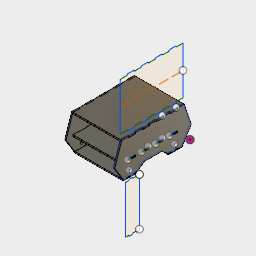
Phantom Chassis v1 (Autodesk Fusion 360 design; units mm, degrees)
Autodesk Fusion 360 part; units mm, degrees
note: some values were not read from the file. Set by a fixed rule: which sketch regions a step uses.
sketch "Sketch1" plane through (0, 0, 0) normal (1, 0, 0) x (0, 1, 0)
  line L0 (-200, 100) -> (-220, 40)
  line L1 (-195, 0) -> (-220, 40)
  line L2 (-25, 0) -> (0, 40)
  line L3 (0, 40) -> (-20, 100)
  line L4 (-65, 0) -> (-85, 15)
  line L5 (-85, 15) -> (-135, 15)
  line L6 (-135, 15) -> (-155, 0)
  line L7 (-179.9981, 100) -> (-179.9981, 97)
  line L8 (-160, 97) -> (-160, 100)
  line L9 (-179.9981, 100) -> (-179.9981, 97)
  line L10 (-160, 97) -> (-160, 100)
  line L11 (-160, 100) -> (-140, 100)
  line L12 (-140, 100) -> (-140, 97)
  line L13 (-20, 100) -> (-40, 100)
  line L14 (-40, 100) -> (-40, 97)
  line L15 (-60, 97) -> (-60, 100)
  line L16 (-40, 100) -> (-40, 97)
  line L17 (-60, 100) -> (-80, 100)
  line L18 (-80, 100) -> (-80, 97)
  line L19 (-60, 97) -> (-60, 100)
  line L20 (-140, 97) -> (-140, 100)
  line L21 (-80, 100) -> (-80, 97)
  line L22 (-40, 100) -> (-20, 100)
  line L23 (-80, 100) -> (-60, 100)
  line L24 (-200, 100) -> (-179.9981, 100)
  line L25 (-160, 100) -> (-140, 100)
  line L26 (-160, 97) -> (-179.9981, 97)
  line L27 (-40, 97) -> (-60, 97)
  line L28 (-120, 96.9801) -> (-120, 100)
  line L29 (-120, 96.9801) -> (-140, 97)
  line L30 (-65, 0) -> (-55, 0)
  line L31 (-25, 0) -> (-25, -3)
  line L32 (-25, -3) -> (-35, -3)
  line L33 (-35, 0) -> (-35, -3)
  line L34 (-45, -3) -> (-45, 0)
  line L35 (-55, -3) -> (-55, 0)
  line L36 (-35, 0) -> (-45, 0)
  line L37 (-55, 0) -> (-65, 0)
  line L38 (-35, 0) -> (-45, 0)
  line L39 (-55, 0) -> (-65, 0)
  line L40 (-55, -3) -> (-45, -3)
  line L41 (-195, 0) -> (-195, -3)
  line L42 (-195, -3) -> (-185, -3)
  line L43 (-185, -3) -> (-185, 0)
  line L44 (-175, 0) -> (-175, -3)
  line L45 (-175, -3) -> (-165, -3)
  line L46 (-165, -3) -> (-165, 0)
  line L47 (-180, 40) -> (-180, 43)
  line L48 (-140, 43) -> (-140, 40)
  line L49 (-100, 43) -> (-100, 40)
  line L50 (-120, 40) -> (-120, 44)
  line L51 (-60, 43) -> (-60, 40)
  line L52 (-80, 40) -> (-80, 44)
  line L53 (-40, 43) -> (-40, 40)
  line L54 (-155, 0) -> (-165, 0)
  line L55 (-175, 0) -> (-185, 0)
  line L56 (-185, 0) -> (-175, 0)
  line L57 (-165, 0) -> (-155, 0)
  line L58 (-120, 100) -> (-100, 100)
  line L59 (-80, 97) -> (-100, 97)
  line L60 (-100, 97) -> (-100, 100)
  line L61 (-180, 43) -> (-160, 43)
  line L62 (-160, 43) -> (-160, 40)
  line L63 (-160, 40) -> (-180, 40)
  line L64 (-180, 40) -> (-180, 43)
  line L65 (-140, 43) -> (-120, 43)
  line L66 (-120, 43) -> (-120, 40)
  line L67 (-120, 40) -> (-140, 40)
  line L68 (-140, 40) -> (-140, 43)
  line L69 (-100, 43) -> (-80, 43)
  line L70 (-80, 43) -> (-80, 40)
  line L71 (-80, 40) -> (-100, 40)
  line L72 (-100, 40) -> (-100, 43)
  line L73 (-60, 43) -> (-40, 43)
  line L74 (-40, 43) -> (-40, 40)
  line L75 (-40, 40) -> (-60, 40)
  line L76 (-60, 40) -> (-60, 43)
  circle A0 centre (-175, 12) radius 4
  circle A1 centre (-45, 12) radius 4
  dimension "d22" = 3
  dimension "d23" = 3
  dimension "d25" = 3
  dimension "d26" = 3
  dimension "d27" = 3
  dimension "d28" = 3
  dimension "d29" = 3
  dimension "d30" = 3
  dimension "d42" = 3
  constraint horizontal L24
  constraint coincident origin L24
  constraint coincident origin L38
  constraint vertical L7
  constraint vertical L8
  constraint vertical L9
  constraint vertical L10
  constraint horizontal L11
  constraint vertical L12
  constraint vertical L14
  constraint vertical L15
  constraint vertical L16
  constraint vertical L19
  constraint vertical L20
  constraint collinear L24 L25
  constraint coincident L27
  constraint perpendicular L31 L32
  constraint perpendicular L32 L33
  constraint perpendicular L34 L36
  constraint perpendicular L33 L38
  constraint perpendicular L34 L40
  constraint perpendicular L41 L54
  constraint perpendicular L41 L42
  constraint coincident origin L54
  constraint perpendicular L44 L54
  constraint perpendicular L44 L45
  constraint coincident origin L56
  constraint vertical L47
  constraint vertical L48
  constraint vertical L49
  constraint vertical L50
  constraint vertical L51
  constraint vertical L52
  constraint vertical L53
  constraint collinear L54 L55
  constraint collinear L56 L57
  constraint perpendicular L28 L58
  constraint perpendicular L18 L59
  constraint perpendicular L58 L60
  constraint horizontal L61
  constraint vertical L62
  constraint horizontal L63
  constraint vertical L64
  constraint horizontal L65
  constraint vertical L66
  constraint horizontal L67
  constraint vertical L68
  constraint horizontal L69
  constraint vertical L70
  constraint horizontal L71
  constraint vertical L72
  constraint horizontal L73
  constraint vertical L74
  constraint horizontal L75
  constraint vertical L76
  constraint perpendicular L30 L35
  constraint collinear L17 L58
  constraint collinear L13 L17
  measures "d42" distance of origin
sketch "Sketch3" plane through (0, 0, 0) normal (1, 0, 0) x (0, 1, 0)
  line L0 (-175, -11) -> (-165, -11)
  line L1 (-165, -11) -> (-165, -14)
  line L2 (-175, -14) -> (-175, -11)
  line L3 (-155, -11) -> (-145, -11)
  line L4 (-145, -11) -> (-145, -14)
  line L5 (-155, -14) -> (-155, -11)
  line L6 (-145, -14) -> (-145, -153)
  line L7 (-185, -150) -> (-185, -14)
  line L8 (-175, -153) -> (-165, -153)
  line L9 (-165, -153) -> (-165, -150)
  line L10 (-175, -150) -> (-175, -153)
  line L11 (-145, -150) -> (-145, -153)
  line L12 (-145, -153) -> (-155, -153)
  line L13 (-155, -153) -> (-155, -150)
  line L14 (-175, -150) -> (-185, -150)
  line L15 (-165, -150) -> (-155, -150)
  line L16 (-145, -153) -> (-155, -153)
  line L17 (-165, -153) -> (-175, -153)
  line L18 (-185, -14) -> (-175, -14)
  line L19 (-165, -14) -> (-155, -14)
  dimension "d39" = 3
  dimension "d40" = 3
  dimension "d41" = 3
  constraint horizontal L0
  constraint vertical L1
  constraint vertical L2
  constraint horizontal L3
  constraint vertical L4
  constraint vertical L5
  constraint horizontal L18
  constraint vertical L6
  constraint horizontal L16
  constraint vertical L7
  constraint horizontal L8
  constraint vertical L9
  constraint vertical L10
  constraint vertical L11
  constraint horizontal L12
  constraint vertical L13
  constraint perpendicular L7 L14
  constraint perpendicular L9 L15
  constraint collinear L16 L17
  constraint collinear L18 L19
sketch "Sketch4" plane through (0, 0, 0) normal (1, 0, 0) x (0, 1, 0)
  line L0 (-20, 115) -> (-20, 250)
  line L1 (-40, 111) -> (-60, 111)
  line L2 (-60, 111) -> (-40, 111)
  line L3 (-20, 114) -> (-20, 115)
  line L4 (-20, 114) -> (-40, 114)
  line L5 (-40, 114) -> (-40, 111)
  line L6 (-60, 111) -> (-60, 114)
  line L7 (-60, 114) -> (-80, 114)
  line L8 (-80, 114) -> (-80, 111)
  line L9 (-80, 111) -> (-100, 111)
  line L10 (-100, 111) -> (-100, 114)
  line L11 (-100, 114) -> (-120, 114)
  line L12 (-120, 114) -> (-120, 111)
  line L13 (-120, 111) -> (-140, 111)
  line L14 (-140, 111) -> (-140, 114)
  line L15 (-140, 114) -> (-160, 114)
  line L16 (-160, 114) -> (-160, 111)
  line L17 (-160, 111) -> (-180, 111)
  line L18 (-180, 111) -> (-180, 114)
  line L19 (-180, 114) -> (-200, 114)
  line L20 (-200, 114) -> (-200, 250)
  line L21 (-20, 250) -> (-40, 250)
  line L22 (-40, 250) -> (-40, 253)
  line L23 (-40, 253) -> (-60, 253)
  line L24 (-60, 253) -> (-60, 250)
  line L25 (-60, 250) -> (-80, 250)
  line L26 (-80, 250) -> (-80, 253)
  line L27 (-80, 253) -> (-100, 253)
  line L28 (-100, 253) -> (-100, 250)
  line L29 (-100, 250) -> (-120, 250)
  line L30 (-120, 250) -> (-120, 253)
  line L31 (-120, 253) -> (-140, 253)
  line L32 (-140, 253) -> (-140, 250)
  line L33 (-140, 250) -> (-160, 250)
  line L34 (-160, 250) -> (-160, 253)
  line L35 (-160, 253) -> (-180, 253)
  line L36 (-180, 253) -> (-180, 250)
  line L37 (-180, 250) -> (-200, 250)
  line L38 (-200, 182) -> (-20, 182) construction
  dimension "d31" = 3
  dimension "d32" = 3
  dimension "d33" = 3
  dimension "d34" = 3
  dimension "d35" = 3
  dimension "d36" = 3
  dimension "d37" = 3
  dimension "d38" = 3
  constraint vertical L0
  constraint horizontal L1
  constraint parallel L0 L3
  constraint perpendicular L3 L4
  constraint perpendicular L1 L5
  constraint perpendicular L1 L6
  constraint perpendicular L6 L7
  constraint parallel L6 L8
  constraint perpendicular L8 L9
  constraint perpendicular L9 L10
  constraint perpendicular L10 L11
  constraint perpendicular L11 L12
  constraint perpendicular L12 L13
  constraint perpendicular L13 L14
  constraint perpendicular L14 L15
  constraint perpendicular L15 L16
  constraint perpendicular L14 L17
  constraint perpendicular L17 L18
  constraint perpendicular L19 L20
  constraint perpendicular L0 L21
  constraint perpendicular L21 L22
  constraint perpendicular L22 L23
  constraint perpendicular L21 L24
  constraint perpendicular L22 L25
  constraint perpendicular L21 L26
  constraint perpendicular L26 L27
  constraint perpendicular L27 L28
  constraint perpendicular L28 L29
  constraint perpendicular L29 L30
  constraint perpendicular L30 L31
  constraint perpendicular L31 L32
  constraint perpendicular L32 L33
  constraint perpendicular L33 L34
  constraint perpendicular L32 L35
  constraint perpendicular L35 L36
  constraint perpendicular L20 L37
  constraint midpoint L20 origin
  measures "d31" distance of origin
  measures "d32" distance of origin
  measures "d33" distance of origin
  measures "d34" distance of origin
  measures "d35" distance of origin
  measures "d36" distance of origin
  measures "d37" distance of origin
  measures "d38" distance of origin
extrude "Extrude1" add sketch "Sketch4" along normal blind 4 makes body 1
extrude "Extrude2" add sketch "Sketch1" along normal blind 4 separate body makes body 2
extrude "Extrude3" add sketch "Sketch3" along normal blind 4 separate body makes body 3
extrude "Extrude4" add sketch "Sketch4" along normal blind 4 separate body makes body 4
extrude "Extrude5" add sketch "Sketch1" along normal blind 4 separate body makes body 5
extrude "Extrude6" add sketch "Sketch3" along normal blind 4 separate body makes body 6
move_body "MoveBody1" bodies 4 to x (0, 0, 1) y (0, 1, 0) z (-1, 0, 0) at (157.1293, 0, 157.1293)
move_body "MoveBody2" bodies 1 to x (0, 0, -1) y (0, 1, 0) z (1, 0, 0) at (-198.7281, 0, 206.7281)
move_body "MoveBody3" bodies 6 to x (0, 0, -1) y (0, 1, 0) z (1, 0, 0) at (44.7719, 0, -44.7719)
move_body "MoveBody4" bodies 3 to x (0, 0, -1) y (0, 1, 0) z (1, 0, 0) at (91.1516, 0, -91.1516)
move_body "MoveBody5" bodies 6 to x (1, 0, 0) y (0, 1, 0) z (0, 0, 1) at (0, -10, 45)
move_body "MoveBody6" bodies 6 to x (1, 0, 0) y (0, 1, 0) z (0, 0, 1) at (0, 0, -0.25)
move_body "MoveBody7" bodies 6 to x (1, 0, 0) y (0, 1, 0) z (0, 0, 1) at (-30.8, 0, 0)
move_body "MoveBody8" bodies 4 to x (1, 0, 0) y (0, 1, 0) z (0, 0, 1) at (-43, 0, -117)
move_body "MoveBody9" bodies 3 to x (1, 0, 0) y (0, 1, 0) z (0, 0, 1) at (-77.2, 0, 90)
move_body "MoveBody10" bodies 3 to x (1, 0, 0) y (0, 1, 0) z (0, 0, 1) at (0, 0, 1.1)
move_body "MoveBody11" bodies 3 to x (1, 0, 0) y (0, 1, 0) z (0, 0, 1) at (0, 120, 0)
move_body "MoveBody12" bodies 3 to x (1, 0, 0) y (0, 1, 0) z (0, 0, 1) at (0, 0, 0.05)
move_body "MoveBody13" bodies 3 to x (1, 0, 0) y (0, 1, 0) z (0, 0, 1) at (0.05, 0, 0)
move_body "MoveBody14" bodies 6 to x (1, 0, 0) y (0, 1, 0) z (0, 0, 1) at (0, 0, 0.02)
move_body "MoveBody15" bodies 5 to x (1, 0, 0) y (0, 1, 0) z (0, 0, 1) at (-140.05, 0, 0)
move_body "MoveBody16" bodies 1 to x (1, 0, 0) y (0, 1, 0) z (0, 0, 1) at (-51.2, 0, -106.7)
move_body "MoveBody17" bodies 3 to x (1, 0, 0) y (0, -1, 0) z (0, 0, -1) at (0, -116.1802, -8.0033)
move_body "MoveBody18" bodies 3 to x (1, 0, 0) y (0, 1, 0) z (0, 0, 1) at (0, 26, 4)
move_body "MoveBody19" bodies 3 to x (1, 0, 0) y (0, 1, 0) z (0, 0, 1) at (0, 0.2, 0)
move_body "MoveBody20" bodies 5 to x (1, 0, 0) y (0, 1, 0) z (0, 0, 1) at (0.12, 0, 0.04)
move_body "MoveBody21" bodies 6 to x (1, 0, 0) y (0, 1, 0) z (0, 0, 1) at (0.1, 0, 0.05)
move_body "MoveBody22" bodies 6 to x (1, 0, 0) y (0, 1, 0) z (0, 0, 1) at (0, 0, -0.01)
move_body "MoveBody23" bodies 3 to x (1, 0, 0) y (0, 1, 0) z (0, 0, 1) at (0.07, 0, 0)
move_body "MoveBody24" bodies 3 to x (1, 0, 0) y (0, 1, 0) z (0, 0, 1) at (0, 0, 0.04)
move_body "MoveBody25" bodies 2 to x (1, 0, 0) y (0, 1, 0) z (0, 0, 1) at (0.07, 0, 0)
move_body "MoveBody26" bodies 2 to x (1, 0, 0) y (0, 1, 0) z (0, 0, 1) at (0.002, 0, 0)
move_body "MoveBody27" bodies 2 to x (1, 0, 0) y (0, 1, 0) z (0, 0, 1) at (0, 0, 0.038)
equation "thick = 3 mm"
equation "d22 = thick"
equation "d23 = thick"
equation "d25 = thick"
equation "d26 = thick"
equation "d27 = thick"
equation "d28 = thick"
equation "d29 = thick"
equation "d30 = thick"
equation "d31 = thick"
equation "d32 = thick"
equation "d33 = thick"
equation "d34 = thick"
equation "d35 = thick"
equation "d36 = thick"
equation "d37 = thick"
equation "d38 = thick"
equation "d39 = thick"
equation "d40 = thick"
equation "d41 = thick"
equation "d42 = thick"
